Autodesk Fusion 360 part; units mm, degrees
(part 13 of 24)
  arc A3081 (7.8145, 16.0591) -> (7.8145, 16.3766) centre (7.8145, 16.2179) ccw
  arc A3082 (12.5666, 11.6245) -> (12.2491, 11.6245) centre (12.4078, 11.6245) ccw
  line L1039 (15.6337, 7.0391) -> (14.6591, 8.0137)
  line L1040 (12.4079, 11.6245) -> (12.259, 11.9839)
  arc A3083 (3.7529, 15.8555) -> (3.4354, 15.8555) centre (3.5941, 15.8555) ccw
  line L1041 (10.4521, 11.0249) -> (10.4521, 8.6955)
  arc A3084 (10.6108, 11.0249) -> (10.2934, 11.0249) centre (10.4521, 11.0249) ccw
  arc A3085 (10.4543, 8.2753) -> (10.7476, 8.3968) centre (10.601, 8.3361) ccw
  arc A3086 (72.6868, 22.0663) -> (72.6868, 22.3838) centre (72.6868, 22.2251) ccw
  arc A3087 (5.6955, 13.5954) -> (5.6955, 13.9129) centre (5.6955, 13.7542) ccw
  arc A3088 (14.3009, 32.0866) -> (14.3009, 32.404) centre (14.3009, 32.2453) ccw
  arc A3089 (56.8579, 22.3838) -> (56.8579, 22.0663) centre (56.8579, 22.2251) ccw
  arc A3090 (15.3797, 3.6512) -> (15.3797, 3.9687) centre (15.3797, 3.81) ccw
  arc A3091 (7.2149, 14.1034) -> (7.2149, 14.4208) centre (7.2149, 14.2621) ccw
  arc A3092 (14.5539, 2.2416) -> (14.5539, 2.5591) centre (14.5539, 2.4004) ccw
  arc A3093 (4.4645, 16.8846) -> (4.4645, 16.5671) centre (4.4645, 16.7259) ccw
  arc A3094 (15.7924, 7.0391) -> (15.4749, 7.0391) centre (15.6337, 7.0391) ccw
  arc A3095 (14.4417, 2.5126) -> (14.6662, 2.288) centre (14.554, 2.4003) ccw
  arc A3096 (13.8113, 3.81) -> (14.1288, 3.81) centre (13.9701, 3.81) ccw
  arc A3097 (13.8113, 2.4003) -> (14.1288, 2.4003) centre (13.9701, 2.4003) ccw
  line L1042 (13.6391, 32.2453) -> (14.3009, 32.2453)
  arc A3098 (6.2035, 16.3766) -> (6.2035, 16.0591) centre (6.2035, 16.2179) ccw
  line L1043 (3.5941, 14.6245) -> (4.4645, 13.7541)
  arc A3099 (12.1476, 5.6609) -> (12.465, 5.6609) centre (12.3063, 5.6609) ccw
  line L1044 (10.4521, 8.6955) -> (10.601, 8.3361)
  arc A3100 (44.8038, 14.6194) -> (44.5105, 14.7409) centre (44.6572, 14.6802) ccw
  arc A3101 (44.6251, 14.2194) -> (44.3076, 14.2194) centre (44.4664, 14.2194) ccw
  line L1045 (13.6893, 8.0137) -> (12.4079, 9.2951)
  line L1046 (12.5603, 3.2261) -> (13.3861, 2.4003)
  arc A3102 (12.2612, 11.5638) -> (12.5546, 11.6853) centre (12.4079, 11.6246) ccw
  line L1047 (13.0668, 4.9004) -> (12.5603, 4.3939)
  arc A3103 (45.5314, 15.077) -> (45.4099, 15.3704) centre (45.4706, 15.2237) ccw
  arc A3104 (3.4354, 14.6245) -> (3.7529, 14.6245) centre (3.5941, 14.6245) ccw
  line L1048 (44.4663, 13.7206) -> (44.6572, 13.2598)
  arc A3105 (13.6893, 8.1724) -> (13.6893, 7.8549) centre (13.6893, 8.0137) ccw
  arc A3106 (14.7714, 8.126) -> (14.5469, 7.9014) centre (14.6592, 8.0137) ccw
  arc A3107 (12.2491, 9.2951) -> (12.5666, 9.2951) centre (12.4078, 9.2951) ccw
  arc A3108 (6.2035, 14.4208) -> (6.2035, 14.1034) centre (6.2035, 14.2621) ccw
  line L1049 (3.5941, 15.8555) -> (3.5941, 14.6245)
  arc A3109 (8.1132, 15.9224) -> (8.2347, 16.2157) centre (8.1739, 16.0691) ccw
  arc A3110 (6.0912, 16.1056) -> (6.3157, 16.3302) centre (6.2035, 16.2179) ccw
  line L1050 (7.8145, 16.2179) -> (6.2035, 16.2179)
  arc A3111 (4.3523, 13.6418) -> (4.5768, 13.8664) centre (4.4646, 13.7541) ccw
  arc A3112 (12.5202, 9.4073) -> (12.2956, 9.1828) centre (12.4079, 9.2951) ccw
  arc A3113 (12.1468, 11.8717) -> (12.3713, 12.0962) centre (12.2591, 11.984) ccw
  arc A3114 (14.6591, 7.8549) -> (14.6591, 8.1724) centre (14.6591, 8.0137) ccw
  arc A3115 (7.8753, 16.3646) -> (7.7538, 16.0712) centre (7.8146, 16.2179) ccw
  arc A3116 (4.5768, 16.6136) -> (4.3523, 16.8382) centre (4.4645, 16.7259) ccw
  arc A3117 (10.3398, 10.9127) -> (10.5644, 11.1372) centre (10.4521, 11.025) ccw
  arc A3118 (5.6955, 16.5671) -> (5.6955, 16.8846) centre (5.6955, 16.7259) ccw
  line L1051 (14.6591, 8.0137) -> (13.6893, 8.0137)
  arc A3119 (5.5832, 13.8664) -> (5.8077, 13.6418) centre (5.6954, 13.7541) ccw
  arc A3120 (44.3076, 13.7206) -> (44.6251, 13.7206) centre (44.4664, 13.7206) ccw
  arc A3121 (44.3196, 14.2801) -> (44.613, 14.1586) centre (44.4663, 14.2193) ccw
  line L1052 (5.6955, 16.7259) -> (4.4645, 16.7259)
  arc A3122 (3.4818, 15.9677) -> (3.7064, 15.7432) centre (3.5941, 15.8554) ccw
  line L1053 (12.259, 11.9839) -> (11.9839, 12.259)
  arc A3123 (3.7064, 14.7368) -> (3.4818, 14.5123) centre (3.5941, 14.6246) ccw
  line L1054 (45.4706, 15.2237) -> (45.0098, 15.0328)
  arc A3124 (12.4057, 12.0447) -> (12.1124, 11.9232) centre (12.2591, 11.984) ccw
  arc A3125 (12.4016, 3.81) -> (12.719, 3.81) centre (12.5603, 3.81) ccw
  arc A3126 (14.1287, 3.81) -> (13.8112, 3.81) centre (13.97, 3.81) ccw
  line L1055 (12.5603, 3.81) -> (13.97, 3.81)
  line L1056 (5.6955, 13.7541) -> (6.2035, 14.2621)
  arc A3127 (5.8077, 16.8382) -> (5.5832, 16.6136) centre (5.6954, 16.7259) ccw
  line L1057 (12.3063, 5.6609) -> (13.0668, 4.9004)
  line L1058 (12.5603, 4.3939) -> (12.5603, 3.81)
  line L1059 (6.2035, 14.2621) -> (7.2149, 14.2621)
  line L1060 (8.1739, 16.069) -> (7.8145, 16.2179)
  arc A3128 (6.3157, 14.1498) -> (6.0912, 14.3744) centre (6.2035, 14.2621) ccw
  line L1061 (44.6572, 13.2598) -> (44.7421, 13.1749)
  line L1062 (10.601, 8.3361) -> (12.3063, 6.6307)
  arc A3129 (44.5105, 13.1991) -> (44.8038, 13.3206) centre (44.6572, 13.2599) ccw
  arc A3130 (10.2934, 8.6955) -> (10.6108, 8.6955) centre (10.4521, 8.6955) ccw
  line L1063 (11.9839, 12.259) -> (8.1739, 16.069)
  arc A3131 (12.4016, 3.2261) -> (12.719, 3.2261) centre (12.5603, 3.2261) ccw
  line L1064 (4.4645, 16.7259) -> (3.5941, 15.8555)
  arc A3132 (15.5214, 6.9269) -> (15.746, 7.1514) centre (15.6337, 7.0391) ccw
  arc A3133 (13.577, 7.9014) -> (13.8015, 8.1259) centre (13.6893, 8.0137) ccw
  arc A3134 (12.5603, 3.9688) -> (12.5603, 3.6513) centre (12.5603, 3.81) ccw
  arc A3135 (46.8149, 13.7206) -> (47.1324, 13.7206) centre (46.9737, 13.7206) ccw
  arc A3136 (12.194, 6.5185) -> (12.4186, 6.743) centre (12.3063, 6.6308) ccw
  arc A3137 (44.7694, 13.3721) -> (44.5449, 13.1476) centre (44.6571, 13.2599) ccw
  arc A3138 (12.465, 6.6307) -> (12.1476, 6.6307) centre (12.3063, 6.6307) ccw
  arc A3139 (44.6298, 13.0626) -> (44.8544, 13.2872) centre (44.7421, 13.1749) ccw
  line L1065 (44.7421, 13.1749) -> (44.7421, 7.8557)
  arc A3140 (44.8028, 7.709) -> (44.6814, 8.0024) centre (44.7421, 7.8557) ccw
  arc A3141 (44.9008, 13.1749) -> (44.5834, 13.1749) centre (44.7421, 13.1749) ccw
  arc A3142 (45.9694, 15.0649) -> (45.9694, 15.3824) centre (45.9694, 15.2236) ccw
  arc A3143 (13.2738, 2.288) -> (13.4983, 2.5126) centre (13.3861, 2.4003) ccw
  arc A3144 (40.0108, 7.9016) -> (40.1089, 7.5996) centre (40.0599, 7.7506) ccw
  arc A3145 (46.5424, 15.1451) -> (46.3179, 14.9206) centre (46.4301, 15.0329) ccw
  line L1066 (44.6572, 14.6802) -> (44.4663, 14.2194)
  arc A3146 (44.6593, 7.9932) -> (44.7808, 7.6999) centre (44.7201, 7.8466) ccw
  arc A3147 (43.5919, 8.262) -> (43.4704, 7.9686) centre (43.5312, 8.1153) ccw
  arc A3148 (44.1192, 7.6999) -> (44.2407, 7.9932) centre (44.1799, 7.8466) ccw
  arc A3149 (13.179, 4.7881) -> (12.9545, 5.0126) centre (13.0668, 4.9003) ccw
  arc A3150 (43.5311, 7.9565) -> (43.5311, 8.274) centre (43.5311, 8.1152) ccw
  arc A3151 (46.6706, 14.5679) -> (46.8951, 14.7924) centre (46.7829, 14.6801) ccw
  line L1067 (46.4302, 15.0328) -> (45.9694, 15.2237)
  arc A3152 (46.0301, 15.3704) -> (45.9086, 15.077) centre (45.9694, 15.2237) ccw
  line L1068 (45.9694, 15.2237) -> (45.4706, 15.2237)
  arc A3153 (46.9295, 14.7409) -> (46.6362, 14.6194) centre (46.7828, 14.6801) ccw
  arc A3154 (12.719, 4.3939) -> (12.4016, 4.3939) centre (12.5603, 4.3939) ccw
  line L1069 (12.5603, 3.81) -> (12.5603, 3.2261)
  arc A3155 (45.4706, 15.3824) -> (45.4706, 15.0649) centre (45.4706, 15.2236) ccw
  arc A3156 (47.1324, 14.2194) -> (46.8149, 14.2194) centre (46.9737, 14.2194) ccw
  arc A3157 (44.5834, 7.8557) -> (44.9008, 7.8557) centre (44.7421, 7.8557) ccw
  arc A3158 (12.6726, 3.3383) -> (12.448, 3.1138) centre (12.5603, 3.2261) ccw
  arc A3159 (13.97, 3.6513) -> (13.97, 3.9688) centre (13.97, 3.81) ccw
  line L1070 (46.9737, 14.2194) -> (46.7828, 14.6802)
  arc A3160 (46.3694, 14.8862) -> (46.4909, 15.1795) centre (46.4301, 15.0328) ccw
  arc A3161 (44.5449, 14.7924) -> (44.7694, 14.5679) centre (44.6571, 14.6802) ccw
  line L1071 (44.72, 7.8465) -> (44.45, 7.5765)
  line L1072 (44.7421, 7.8557) -> (44.72, 7.8465)
  line L1073 (44.4663, 14.2194) -> (44.4663, 13.7206)
  line L1074 (45.0098, 15.0328) -> (44.6572, 14.6802)
  line L1075 (39.6555, 7.5028) -> (39.4872, 7.3345)
  line L1076 (46.7828, 14.6802) -> (46.4302, 15.0328)
  arc A3162 (44.613, 13.7814) -> (44.3196, 13.6599) centre (44.4663, 13.7206) ccw
  arc A3163 (13.97, 3.6512) -> (13.97, 3.9687) centre (13.97, 3.81) ccw
  arc A3164 (12.4186, 5.7731) -> (12.194, 5.5486) centre (12.3063, 5.6609) ccw
  line L1077 (40.2861, 7.8241) -> (40.0599, 7.7506)
  line L1078 (46.9737, 13.7206) -> (46.9737, 14.2194)
  arc A3165 (41.6181, 7.5092) -> (41.8426, 7.2846) centre (41.7303, 7.3969) ccw
  arc A3166 (45.1221, 14.9206) -> (44.8976, 15.1451) centre (45.0099, 15.0328) ccw
  arc A3167 (39.375, 7.4468) -> (39.5995, 7.2223) centre (39.4873, 7.3346) ccw
  arc A3168 (12.719, 3.81) -> (12.4016, 3.81) centre (12.5603, 3.81) ccw
  arc A3169 (13.8112, 3.81) -> (14.1287, 3.81) centre (13.97, 3.81) ccw
  arc A3170 (40.9691, 7.6673) -> (41.0187, 7.9809) centre (40.9939, 7.8241) ccw
  line L1079 (43.5311, 8.1153) -> (42.8289, 8.1153)
  arc A3171 (42.8896, 7.9686) -> (42.7681, 8.262) centre (42.8289, 8.1153) ccw
  line L1080 (13.97, 3.81) -> (12.5603, 3.81)
  arc A3172 (44.9491, 15.1795) -> (45.0706, 14.8862) centre (45.0099, 15.0328) ccw
  arc A3173 (42.2923, 7.7343) -> (42.0678, 7.9588) centre (42.18, 7.8466) ccw
  arc A3174 (12.9545, 4.7881) -> (13.179, 5.0126) centre (13.0668, 4.9003) ccw
  arc A3175 (40.64, 8.02) -> (40.64, 7.7025) centre (40.64, 7.8613) ccw
  line L1081 (41.2201, 7.7506) -> (40.9939, 7.8241)
  arc A3176 (12.448, 4.5062) -> (12.6726, 4.2817) centre (12.5603, 4.394) ccw
  line L1082 (40.9939, 7.8241) -> (40.7589, 7.8613)
  arc A3177 (46.827, 14.1586) -> (47.1204, 14.2801) centre (46.9737, 14.2194) ccw
  arc A3178 (41.7368, 7.615) -> (41.5123, 7.3905) centre (41.6246, 7.5027) ccw
  arc A3179 (12.5603, 3.9687) -> (12.5603, 3.6512) centre (12.5603, 3.81) ccw
  arc A3180 (39.7677, 7.3905) -> (39.5432, 7.615) centre (39.6555, 7.5028) ccw
  line L1083 (42.8289, 8.1153) -> (42.18, 7.8465)
  arc A3181 (40.7987, 7.8613) -> (40.4812, 7.8613) centre (40.6399, 7.8613) ccw
  arc A3182 (41.5312, 7.3743) -> (41.7179, 7.6312) centre (41.6246, 7.5027) ccw
  arc A3183 (41.36, 7.5011) -> (41.5042, 7.784) centre (41.4321, 7.6425) ccw
  arc A3184 (40.7988, 7.8613) -> (40.4813, 7.8613) centre (40.6401, 7.8613) ccw
  arc A3185 (40.64, 6.1913) -> (40.64, 6.5088) centre (40.64, 6.3501) ccw
  arc A3186 (39.2416, 7.2665) -> (39.4984, 7.0799) centre (39.37, 7.1732) ccw
  arc A3187 (34.6723, 7.7343) -> (34.4478, 7.9588) centre (34.5601, 7.8466) ccw
  arc A3188 (41.043, 7.9751) -> (40.9448, 7.6731) centre (40.9939, 7.8241) ccw
  arc A3189 (38.2438, 8.0181) -> (38.1941, 7.7045) centre (38.2189, 7.8613) ccw
  arc A3190 (41.2922, 7.892) -> (41.1481, 7.6091) centre (41.2202, 7.7506) ccw
  arc A3191 (35.2696, 7.9686) -> (35.1481, 8.262) centre (35.2088, 8.1153) ccw
  line L1084 (40.0599, 7.7506) -> (39.8479, 7.6426)
  arc A3192 (42.8289, 8.274) -> (42.8289, 7.9565) centre (42.8289, 8.1152) ccw
  line L1085 (35.9111, 8.1153) -> (35.2089, 8.1153)
  arc A3193 (38.1, 7.7025) -> (38.1, 8.02) centre (38.1, 7.8613) ccw
  arc A3194 (38.9912, 7.3743) -> (39.1779, 7.6312) centre (39.0846, 7.5028) ccw
  line L1086 (37.7461, 7.8241) -> (37.5199, 7.7506)
  arc A3195 (40.5211, 8.02) -> (40.5211, 7.7025) centre (40.5211, 7.8613) ccw
  arc A3196 (37.2358, 7.784) -> (37.38, 7.5011) centre (37.3079, 7.6425) ccw
  line L1087 (41.7304, 7.3969) -> (41.6245, 7.5028)
  arc A3197 (38.2189, 7.7025) -> (38.2189, 8.02) centre (38.2189, 7.8613) ccw
  line L1088 (37.1155, 7.5028) -> (37.0096, 7.3969)
  arc A3198 (41.6181, 7.2846) -> (41.8426, 7.5092) centre (41.7304, 7.3969) ccw
  line L1089 (39.37, 7.1732) -> (39.2528, 7.3345)
  arc A3199 (38.1, 8.02) -> (38.1, 7.7025) centre (38.1, 7.8613) ccw
  arc A3200 (35.2089, 8.274) -> (35.2089, 7.9565) centre (35.2089, 8.1152) ccw
  line L1090 (39.4872, 7.3345) -> (39.37, 7.1732)
  arc A3201 (37.0221, 7.6312) -> (37.2088, 7.3743) centre (37.1155, 7.5028) ccw
  line L1091 (40.64, 7.8613) -> (40.64, 6.35)
  arc A3202 (38.6311, 7.5996) -> (38.7292, 7.9016) centre (38.6802, 7.7506) ccw
  arc A3203 (40.7838, 8.0181) -> (40.7341, 7.7045) centre (40.7589, 7.8613) ccw
  arc A3204 (36.8973, 7.2846) -> (37.1219, 7.5092) centre (37.0096, 7.3969) ccw
  line L1092 (44.45, 7.5765) -> (44.18, 7.8465)
  line L1093 (39.8479, 7.6426) -> (39.6555, 7.5028)
  arc A3205 (40.1319, 7.6091) -> (39.9878, 7.892) centre (40.0599, 7.7506) ccw
  arc A3206 (40.64, 7.7025) -> (40.64, 8.02) centre (40.64, 7.8613) ccw
  arc A3207 (39.6157, 7.2412) -> (39.3588, 7.4279) centre (39.4873, 7.3346) ccw
  arc A3208 (40.7589, 7.7025) -> (40.7589, 8.02) centre (40.7589, 7.8613) ccw
  line L1094 (40.64, 7.8613) -> (40.5211, 7.8613)
  line L1095 (41.4321, 7.6426) -> (41.2201, 7.7506)
  arc A3209 (39.9412, 7.5141) -> (39.7546, 7.771) centre (39.8479, 7.6425) ccw
  arc A3210 (40.4813, 6.35) -> (40.7988, 6.35) centre (40.6401, 6.35) ccw
  arc A3211 (44.3377, 7.4643) -> (44.5623, 7.6888) centre (44.45, 7.5766) ccw
  line L1096 (41.6245, 7.5028) -> (41.4321, 7.6426)
  arc A3212 (44.3377, 7.6888) -> (44.5623, 7.4643) centre (44.45, 7.5766) ccw
  arc A3213 (40.64, 6.5088) -> (40.64, 6.1913) centre (40.64, 6.3501) ccw
  line L1097 (40.7589, 7.8613) -> (40.64, 7.8613)
  line L1098 (37.9811, 7.8613) -> (37.7461, 7.8241)
  line L1099 (40.5211, 7.8613) -> (40.2861, 7.8241)
  arc A3214 (44.8323, 7.7343) -> (44.6078, 7.9588) centre (44.72, 7.8466) ccw
  arc A3215 (41.5254, 7.771) -> (41.3388, 7.5141) centre (41.4321, 7.6426) ccw
  line L1100 (38.1, 6.35) -> (38.1, 7.8613)
  line L1101 (40.64, 6.35) -> (40.64, 7.8613)
  arc A3216 (40.3352, 7.6731) -> (40.237, 7.9751) centre (40.2861, 7.8241) ccw
  arc A3217 (42.1193, 7.9932) -> (42.2408, 7.6999) centre (42.18, 7.8465) ccw
  arc A3218 (41.1711, 7.5996) -> (41.2692, 7.9016) centre (41.2202, 7.7506) ccw
  line L1102 (44.18, 7.8465) -> (43.5311, 8.1153)
  arc A3219 (40.5459, 7.7045) -> (40.4962, 8.0181) centre (40.5211, 7.8613) ccw
  arc A3220 (44.2922, 7.9588) -> (44.0677, 7.7343) centre (44.18, 7.8465) ccw
  arc A3221 (39.7758, 7.784) -> (39.92, 7.5011) centre (39.8479, 7.6426) ccw
  arc A3222 (34.1777, 7.6888) -> (34.4023, 7.4643) centre (34.29, 7.5765) ccw
  arc A3223 (40.2613, 7.9809) -> (40.3109, 7.6673) centre (40.2861, 7.8241) ccw
  line L1103 (37.5199, 7.7506) -> (37.3079, 7.6426)
  arc A3224 (39.5621, 7.6312) -> (39.7488, 7.3743) centre (39.6555, 7.5028) ccw
  line L1104 (34.56, 7.8465) -> (34.29, 7.5765)
  arc A3225 (40.4812, 6.35) -> (40.7987, 6.35) centre (40.6399, 6.35) ccw
  line L1105 (42.18, 7.8465) -> (41.7304, 7.3969)
  arc A3226 (38.9854, 7.771) -> (38.7988, 7.5141) centre (38.8921, 7.6425) ccw
  arc A3227 (34.4993, 7.9932) -> (34.6208, 7.6999) centre (34.5601, 7.8466) ccw
  arc A3228 (37.4708, 7.9016) -> (37.5689, 7.5996) centre (37.5199, 7.7506) ccw
  arc A3229 (36.4992, 7.6999) -> (36.6207, 7.9932) centre (36.5599, 7.8466) ccw
  arc A3230 (38.7522, 7.892) -> (38.6081, 7.6091) centre (38.6802, 7.7505) ccw
  arc A3231 (38.4291, 7.6673) -> (38.4787, 7.9809) centre (38.4539, 7.8241) ccw
  arc A3232 (36.8973, 7.5092) -> (37.1219, 7.2846) centre (37.0096, 7.3969) ccw
  arc A3233 (37.5919, 7.6091) -> (37.4478, 7.892) centre (37.5199, 7.7506) ccw
  arc A3234 (39.1968, 7.615) -> (38.9723, 7.3905) centre (39.0846, 7.5028) ccw
  line L1106 (38.2189, 7.8613) -> (38.1, 7.8613)
  line L1107 (29.21, 15.2835) -> (29.48, 15.0135)
  arc A3235 (37.7213, 7.9809) -> (37.7709, 7.6673) centre (37.7461, 7.8241) ccw
  arc A3236 (29.3678, 14.9012) -> (29.5923, 15.1257) centre (29.4801, 15.0135) ccw
  line L1108 (31.6665, 7.493) -> (30.9534, 7.493)
  line L1109 (38.1, 7.8613) -> (38.1, 6.35)
  arc A3237 (38.503, 7.9751) -> (38.4048, 7.6731) centre (38.4539, 7.8241) ccw
  arc A3238 (35.9719, 8.262) -> (35.8504, 7.9686) centre (35.9112, 8.1153) ccw
  arc A3239 (37.9811, 8.02) -> (37.9811, 7.7025) centre (37.9811, 7.8613) ccw
  line L1110 (26.4, 15.0135) -> (26.67, 15.2835)
  arc A3240 (25.6904, 14.8914) -> (25.8119, 14.598) centre (25.7512, 14.7447) ccw
  arc A3241 (30.0681, 14.598) -> (30.1896, 14.8914) centre (30.1288, 14.7447) ccw
  arc A3242 (37.9413, 6.35) -> (38.2588, 6.35) centre (38.1, 6.35) ccw
  arc A3243 (39.3812, 7.4279) -> (39.1243, 7.2412) centre (39.2527, 7.3346) ccw
  arc A3244 (37.4012, 7.5141) -> (37.2146, 7.771) centre (37.3079, 7.6425) ccw
  line L1111 (30.1289, 14.7447) -> (30.8311, 14.7447)
  arc A3245 (38.1, 6.5088) -> (38.1, 6.1913) centre (38.1, 6.3501) ccw
  arc A3246 (23.8907, 15.2687) -> (24.1153, 15.0442) centre (24.003, 15.1565) ccw
  arc A3247 (24.2423, 15.3957) -> (24.0177, 15.1712) centre (24.13, 15.2835) ccw
  arc A3248 (34.1777, 7.4643) -> (34.4023, 7.6888) centre (34.29, 7.5765) ccw
  line L1112 (38.4539, 7.8241) -> (38.2189, 7.8613)
  arc A3249 (39.1405, 7.2223) -> (39.365, 7.4468) centre (39.2528, 7.3346) ccw
  arc A3250 (26.7823, 15.1712) -> (26.5577, 15.3957) centre (26.67, 15.2835) ccw
  line L1113 (24.13, 15.2835) -> (24.4, 15.0135)
  line L1114 (25.0489, 14.7447) -> (25.7511, 14.7447)
  line L1115 (39.2528, 7.3345) -> (39.0845, 7.5028)
  arc A3251 (38.2588, 7.8613) -> (37.9413, 7.8613) centre (38.1, 7.8613) ccw
  arc A3252 (25.0489, 14.9034) -> (25.0489, 14.586) centre (25.0489, 14.7447) ccw
  arc A3253 (29.3223, 15.1712) -> (29.0977, 15.3957) centre (29.21, 15.2835) ccw
  arc A3254 (26.2877, 15.1257) -> (26.5122, 14.9012) centre (26.4, 15.0135) ccw
  line L1116 (39.0845, 7.5028) -> (38.8921, 7.6426)
  arc A3255 (29.3223, 15.3957) -> (29.0977, 15.1712) centre (29.21, 15.2834) ccw
  arc A3256 (38.2587, 7.8613) -> (37.9412, 7.8613) centre (38.0999, 7.8613) ccw
  line L1117 (25.7511, 14.7447) -> (26.4, 15.0135)
  line L1118 (37.0096, 7.3969) -> (36.56, 7.8465)
  arc A3257 (29.5408, 15.1601) -> (29.4193, 14.8668) centre (29.4801, 15.0135) ccw
  arc A3258 (31.6665, 7.3342) -> (31.6665, 7.6517) centre (31.6665, 7.493) ccw
  arc A3259 (34.1322, 7.9588) -> (33.9077, 7.7343) centre (34.02, 7.8466) ccw
  line L1119 (36.56, 7.8465) -> (35.9111, 8.1153)
  line L1120 (34.29, 7.5765) -> (34.02, 7.8465)
  arc A3260 (38.1, 6.1913) -> (38.1, 6.5088) centre (38.1, 6.3501) ccw
  line L1121 (28.94, 15.0135) -> (29.21, 15.2835)
  arc A3261 (37.7952, 7.6731) -> (37.697, 7.9751) centre (37.7461, 7.8241) ccw
  arc A3262 (37.9412, 6.35) -> (38.2587, 6.35) centre (38.0999, 6.35) ccw
  arc A3263 (35.9111, 7.9565) -> (35.9111, 8.274) centre (35.9111, 8.1152) ccw
  line L1122 (38.1, 7.8613) -> (37.9811, 7.8613)
  arc A3264 (37.2277, 7.3905) -> (37.0032, 7.615) centre (37.1155, 7.5028) ccw
  line L1123 (35.2089, 8.1153) -> (34.56, 7.8465)
  arc A3265 (38.0059, 7.7045) -> (37.9562, 8.0181) centre (37.9811, 7.8613) ccw
  line L1124 (38.6801, 7.7506) -> (38.4539, 7.8241)
  arc A3266 (36.6722, 7.9588) -> (36.4477, 7.7343) centre (36.56, 7.8466) ccw
  line L1125 (38.8921, 7.6426) -> (38.6801, 7.7506)
  line L1126 (37.3079, 7.6426) -> (37.1155, 7.5028)
  arc A3267 (38.82, 7.5011) -> (38.9642, 7.784) centre (38.8921, 7.6425) ccw
  arc A3268 (39.2416, 7.0799) -> (39.4984, 7.2665) centre (39.37, 7.1732) ccw
  line L1127 (29.48, 15.0135) -> (30.1289, 14.7447)
  arc A3269 (24.2423, 15.1712) -> (24.0177, 15.3957) centre (24.13, 15.2835) ccw
  arc A3270 (31.5542, 7.6052) -> (31.7787, 7.3807) centre (31.6665, 7.493) ccw
  line L1128 (40.0599, 15.1094) -> (40.2861, 15.0359)
  arc A3271 (29.0007, 14.8668) -> (28.8792, 15.1601) centre (28.94, 15.0135) ccw
  line L1129 (39.8479, 15.2174) -> (40.0599, 15.1094)
  line L1130 (37.7489, 14.7447) -> (38.4511, 14.7447)
  arc A3272 (32.7296, 7.9686) -> (32.6081, 8.262) centre (32.6689, 8.1153) ccw
  arc A3273 (27.5889, 14.9034) -> (27.5889, 14.586) centre (27.5889, 14.7447) ccw
  line L1131 (24.003, 15.1565) -> (24.13, 15.2835)
  line L1132 (32.02, 7.8465) -> (31.6665, 7.493)
  arc A3274 (24.1153, 14.5557) -> (23.8907, 14.3312) centre (24.003, 14.4435) ccw
  line L1133 (30.9534, 7.493) -> (24.003, 14.4434)
  arc A3275 (25.7511, 14.586) -> (25.7511, 14.9034) centre (25.7511, 14.7447) ccw
  arc A3276 (33.4319, 8.262) -> (33.3104, 7.9686) centre (33.3712, 8.1153) ccw
  line L1134 (27.5889, 14.7447) -> (28.2911, 14.7447)
  arc A3277 (23.8442, 14.4434) -> (24.1617, 14.4434) centre (24.003, 14.4434) ccw
  arc A3278 (40.237, 14.8849) -> (40.3352, 15.1869) centre (40.2861, 15.0359) ccw
  arc A3279 (33.3711, 7.9565) -> (33.3711, 8.274) centre (33.3711, 8.1152) ccw
  arc A3280 (34.0807, 14.8668) -> (33.9592, 15.1601) centre (34.02, 15.0135) ccw
  arc A3281 (33.9077, 15.1257) -> (34.1322, 14.9012) centre (34.02, 15.0135) ccw
  arc A3282 (32.1323, 7.7343) -> (31.9078, 7.9588) centre (32.0201, 7.8466) ccw
  arc A3283 (34.6208, 15.1601) -> (34.4993, 14.8668) centre (34.5601, 15.0135) ccw
  line L1135 (34.02, 7.8465) -> (33.3711, 8.1153)
  line L1136 (34.02, 15.0135) -> (34.29, 15.2835)
  line L1137 (24.4, 15.0135) -> (25.0489, 14.7447)
  arc A3284 (26.8278, 14.9012) -> (27.0523, 15.1257) centre (26.9401, 15.0135) ccw
  arc A3285 (30.1289, 14.9034) -> (30.1289, 14.586) centre (30.1289, 14.7447) ccw
  arc A3286 (28.2911, 14.586) -> (28.2911, 14.9034) centre (28.2911, 14.7447) ccw
  arc A3287 (28.2304, 14.8914) -> (28.3519, 14.598) centre (28.2911, 14.7447) ccw
  arc A3288 (39.6619, 15.5753) -> (39.4373, 15.3508) centre (39.5496, 15.4631) ccw
  arc A3289 (34.4023, 15.3957) -> (34.1777, 15.1712) centre (34.29, 15.2834) ccw
  arc A3290 (26.4607, 14.8668) -> (26.3392, 15.1601) centre (26.4, 15.0134) ccw
  arc A3291 (26.7823, 15.3957) -> (26.5577, 15.1712) centre (26.67, 15.2835) ccw
  line L1138 (36.83, 15.2835) -> (37.1, 15.0135)
  arc A3292 (33.3104, 14.8914) -> (33.4319, 14.598) centre (33.3712, 14.7447) ccw
  line L1139 (36.56, 15.0135) -> (36.83, 15.2835)
  arc A3293 (31.3677, 15.1257) -> (31.5922, 14.9012) centre (31.4799, 15.0135) ccw
  arc A3294 (32.6689, 8.274) -> (32.6689, 7.9565) centre (32.6689, 8.1152) ccw
  arc A3295 (39.1607, 14.8668) -> (39.0392, 15.1601) centre (39.1, 15.0135) ccw
  arc A3296 (35.2089, 14.9034) -> (35.2089, 14.586) centre (35.2089, 14.7447) ccw
  arc A3297 (24.4608, 15.1601) -> (24.3393, 14.8668) centre (24.4001, 15.0135) ccw
  arc A3298 (27.0008, 15.1601) -> (26.8793, 14.8668) centre (26.9401, 15.0135) ccw
  arc A3299 (31.9593, 7.9932) -> (32.0808, 7.6999) centre (32.0201, 7.8466) ccw
  arc A3300 (27.5281, 14.598) -> (27.6496, 14.8914) centre (27.5889, 14.7447) ccw
  arc A3301 (30.8311, 14.586) -> (30.8311, 14.9034) centre (30.8311, 14.7447) ccw
  line L1140 (39.6555, 15.3572) -> (39.8479, 15.2174)
  arc A3302 (30.9534, 7.6517) -> (30.9534, 7.3342) centre (30.9534, 7.493) ccw
  line L1141 (24.003, 14.4434) -> (24.003, 15.1565)
  arc A3303 (39.9878, 14.968) -> (40.1319, 15.2509) centre (40.0599, 15.1094) ccw
  line L1142 (26.94, 15.0135) -> (27.5889, 14.7447)
  arc A3304 (36.9423, 15.1712) -> (36.7177, 15.3957) centre (36.83, 15.2835) ccw
  arc A3305 (37.7489, 14.9034) -> (37.7489, 14.586) centre (37.7489, 14.7447) ccw
  arc A3306 (39.92, 15.3589) -> (39.7758, 15.076) centre (39.8479, 15.2175) ccw
  arc A3307 (28.8277, 15.1257) -> (29.0522, 14.9012) centre (28.94, 15.0135) ccw
  arc A3308 (33.9592, 7.6999) -> (34.0807, 7.9932) centre (34.02, 7.8466) ccw
  arc A3309 (24.1617, 15.1565) -> (23.8442, 15.1565) centre (24.003, 15.1565) ccw
  line L1143 (26.67, 15.2835) -> (26.94, 15.0135)
  arc A3310 (30.8412, 7.3807) -> (31.0657, 7.6053) centre (30.9534, 7.493) ccw
  line L1144 (28.2911, 14.7447) -> (28.94, 15.0135)
  line L1145 (32.6689, 8.1153) -> (32.02, 7.8465)
  arc A3311 (39.7488, 15.4857) -> (39.5621, 15.2288) centre (39.6555, 15.3573) ccw
  line L1146 (33.3711, 8.1153) -> (32.6689, 8.1153)
  arc A3312 (24.2878, 14.9012) -> (24.5123, 15.1257) centre (24.4001, 15.0135) ccw
  arc A3313 (24.9881, 14.598) -> (25.1096, 14.8914) centre (25.0489, 14.7447) ccw
  line L1147 (31.75, 15.2835) -> (32.02, 15.0135)
  line L1148 (35.9111, 14.7447) -> (36.56, 15.0135)
  arc A3314 (30.7704, 14.8914) -> (30.8919, 14.598) centre (30.8312, 14.7447) ccw
  line L1149 (32.02, 15.0135) -> (32.6689, 14.7447)
  arc A3315 (36.9878, 14.9012) -> (37.2123, 15.1257) centre (37.1001, 15.0135) ccw
  arc A3316 (32.6689, 14.9034) -> (32.6689, 14.586) centre (32.6689, 14.7447) ccw
  arc A3317 (31.5407, 14.8668) -> (31.4192, 15.1601) centre (31.4799, 15.0135) ccw
  line L1150 (39.5496, 15.4631) -> (39.6555, 15.3572)
  line L1151 (34.56, 15.0135) -> (35.2089, 14.7447)
  arc A3318 (36.4477, 15.1257) -> (36.6722, 14.9012) centre (36.56, 15.0135) ccw
  line L1152 (33.3711, 14.7447) -> (34.02, 15.0135)
  arc A3319 (31.8623, 15.3957) -> (31.6377, 15.1712) centre (31.75, 15.2835) ccw
  line L1153 (40.2861, 15.0359) -> (40.5211, 14.9987)
  arc A3320 (36.9423, 15.3957) -> (36.7177, 15.1712) centre (36.83, 15.2834) ccw
  arc A3321 (35.9111, 14.586) -> (35.9111, 14.9034) centre (35.9111, 14.7447) ccw
  arc A3322 (32.6081, 14.598) -> (32.7296, 14.8914) centre (32.6689, 14.7447) ccw
  line L1154 (35.2089, 14.7447) -> (35.9111, 14.7447)
  line L1155 (31.48, 15.0135) -> (31.75, 15.2835)
  arc A3323 (32.0808, 15.1601) -> (31.9593, 14.8668) centre (32.0201, 15.0134) ccw
  line L1156 (39.1, 15.0135) -> (39.5496, 15.4631)
  arc A3324 (38.9877, 15.1257) -> (39.2122, 14.9012) centre (39.1, 15.0135) ccw
  arc A3325 (39.5432, 15.245) -> (39.7677, 15.4695) centre (39.6555, 15.3573) ccw
  arc A3326 (37.6881, 14.598) -> (37.8096, 14.8914) centre (37.7489, 14.7447) ccw
  arc A3327 (31.8623, 15.1712) -> (31.6377, 15.3957) centre (31.75, 15.2835) ccw
  arc A3328 (31.9078, 14.9012) -> (32.1323, 15.1257) centre (32.0201, 15.0135) ccw
  line L1157 (40.64, 14.9987) -> (40.64, 16.51)
  arc A3329 (41.8896, 15.9789) -> (42.1916, 15.8808) centre (42.0406, 15.9299) ccw
  arc A3330 (38.3904, 14.8914) -> (38.5119, 14.598) centre (38.4511, 14.7447) ccw
  arc A3331 (41.5123, 15.4695) -> (41.7368, 15.245) centre (41.6246, 15.3573) ccw
  arc A3332 (39.7546, 15.089) -> (39.9412, 15.3458) centre (39.8479, 15.2174) ccw
  arc A3333 (38.4511, 14.586) -> (38.4511, 14.9034) centre (38.4511, 14.7447) ccw
  arc A3334 (42.1513, 16.3513) -> (42.1513, 16.6688) centre (42.1513, 16.51) ccw
  line L1158 (30.8311, 14.7447) -> (31.48, 15.0135)
  arc A3335 (40.4962, 14.8419) -> (40.5459, 15.1555) centre (40.5211, 14.9987) ccw
  arc A3336 (40.5211, 15.1574) -> (40.5211, 14.84) centre (40.5211, 14.9987) ccw
  line L1159 (41.7928, 15.5255) -> (41.9326, 15.7179)
  arc A3337 (35.8504, 14.8914) -> (35.9719, 14.598) centre (35.9112, 14.7447) ccw
  line L1160 (42.1141, 16.1561) -> (42.1513, 16.3911)
  arc A3338 (42.31, 16.6289) -> (41.9925, 16.6289) centre (42.1513, 16.6289) ccw
  line L1161 (40.64, 16.51) -> (40.64, 14.9987)
  arc A3339 (39.6619, 15.3508) -> (39.4373, 15.5753) centre (39.5496, 15.4631) ccw
  line L1162 (42.1513, 16.51) -> (42.1513, 16.6289)
  line L1163 (34.29, 15.2835) -> (34.56, 15.0135)
  arc A3340 (33.3711, 14.586) -> (33.3711, 14.9034) centre (33.3711, 14.7447) ccw
  arc A3341 (36.6207, 14.8668) -> (36.4992, 15.1601) centre (36.56, 15.0134) ccw
  line L1164 (37.1, 15.0135) -> (37.7489, 14.7447)
  line L1165 (32.6689, 14.7447) -> (33.3711, 14.7447)
  arc A3342 (37.1608, 15.1601) -> (37.0393, 14.8668) centre (37.1, 15.0134) ccw
  arc A3343 (35.1481, 14.598) -> (35.2696, 14.8914) centre (35.2088, 14.7447) ccw
  arc A3344 (40.1089, 15.2604) -> (40.0108, 14.9584) centre (40.0599, 15.1094) ccw
  line L1166 (38.4511, 14.7447) -> (39.1, 15.0135)
  arc A3345 (34.4478, 14.9012) -> (34.6723, 15.1257) centre (34.5601, 15.0135) ccw
  arc A3346 (40.64, 16.6688) -> (40.64, 16.3513) centre (40.64, 16.51) ccw
  line L1167 (41.2201, 15.1094) -> (41.4321, 15.2174)
  arc A3347 (34.4023, 15.1712) -> (34.1777, 15.3957) centre (34.29, 15.2835) ccw
  arc A3348 (41.9925, 16.51) -> (42.31, 16.51) centre (42.1513, 16.51) ccw
  arc A3349 (40.7987, 16.51) -> (40.4812, 16.51) centre (40.6399, 16.51) ccw
  arc A3350 (41.2692, 14.9584) -> (41.1711, 15.2604) centre (41.2202, 15.1094) ccw
  arc A3351 (40.4813, 16.51) -> (40.7988, 16.51) centre (40.6401, 16.51) ccw
  line L1168 (41.4321, 15.2174) -> (41.6245, 15.3572)
  arc A3352 (40.64, 16.6688) -> (40.64, 16.3513) centre (40.64, 16.51) ccw
  arc A3353 (40.4812, 16.51) -> (40.7987, 16.51) centre (40.6399, 16.51) ccw
  arc A3354 (40.64, 17.8625) -> (40.64, 18.18) centre (40.64, 18.0212) ccw
  arc A3355 (41.9925, 16.3911) -> (42.31, 16.3911) centre (42.1513, 16.3911) ccw
  arc A3356 (40.4812, 14.9987) -> (40.7987, 14.9987) centre (40.6399, 14.9987) ccw
  line L1169 (41.6245, 15.3572) -> (41.7928, 15.5255)
  arc A3357 (41.3388, 15.3458) -> (41.5254, 15.089) centre (41.4321, 15.2174) ccw
  arc A3358 (41.6643, 15.6188) -> (41.9212, 15.4321) centre (41.7927, 15.5255) ccw
  line L1170 (42.0406, 15.9299) -> (42.1141, 16.1561)
  line L1171 (40.9939, 15.0359) -> (41.2201, 15.1094)
  line L1172 (42.0406, 17.0901) -> (41.9326, 17.3021)
  arc A3359 (40.64, 16.6687) -> (40.64, 16.3512) centre (40.64, 16.5099) ccw
  line L1173 (40.2861, 17.9841) -> (40.0599, 17.9106)
  arc A3360 (40.3352, 17.8331) -> (40.237, 18.1351) centre (40.2861, 17.9841) ccw
  arc A3361 (39.7758, 17.944) -> (39.92, 17.6611) centre (39.8479, 17.8026) ccw
  line L1174 (42.1513, 16.51) -> (40.64, 16.51)
  arc A3362 (40.64, 15.1575) -> (40.64, 14.84) centre (40.64, 14.9988) ccw
  arc A3363 (41.9631, 16.8148) -> (42.2651, 16.913) centre (42.1141, 16.8639) ccw
  arc A3364 (39.9412, 17.6741) -> (39.7546, 17.931) centre (39.8479, 17.8025) ccw
  arc A3365 (39.4373, 17.6692) -> (39.6619, 17.4446) centre (39.5496, 17.5569) ccw
  arc A3366 (42.3081, 16.3662) -> (41.9945, 16.4159) centre (42.1513, 16.3911) ccw
  arc A3367 (42.1916, 17.1392) -> (41.8896, 17.0411) centre (42.0406, 17.0902) ccw
  arc A3368 (41.0187, 14.8791) -> (40.9691, 15.1927) centre (40.9939, 15.0359) ccw
  line L1175 (39.1, 18.0065) -> (38.4511, 18.2753)
  line L1176 (41.9326, 15.7179) -> (42.0406, 15.9299)
  arc A3369 (40.1319, 17.7691) -> (39.9878, 18.052) centre (40.0599, 17.9106) ccw
  arc A3370 (41.8041, 17.2088) -> (42.061, 17.3954) centre (41.9326, 17.3021) ccw
  arc A3371 (40.9448, 15.1869) -> (41.043, 14.8849) centre (40.9939, 15.0359) ccw
  line L1177 (40.5211, 18.0213) -> (40.2861, 17.9841)
  arc A3372 (40.7341, 15.1555) -> (40.7838, 14.8419) centre (40.7589, 14.9987) ccw
  arc A3373 (41.905, 15.4132) -> (41.6805, 15.6377) centre (41.7928, 15.5254) ccw
  arc A3374 (40.7988, 16.51) -> (40.4813, 16.51) centre (40.6401, 16.51) ccw
  line L1178 (40.64, 14.9987) -> (40.7589, 14.9987)
  arc A3375 (41.5042, 15.076) -> (41.36, 15.3589) centre (41.4321, 15.2175) ccw
  arc A3376 (42.1513, 16.3512) -> (42.1513, 16.6687) centre (42.1513, 16.5099) ccw
  line L1179 (42.1141, 16.8639) -> (42.0406, 17.0901)
  arc A3377 (42.061, 15.6246) -> (41.8041, 15.8112) centre (41.9326, 15.7179) ccw
  line L1180 (40.64, 16.51) -> (42.1513, 16.51)
  arc A3378 (41.9573, 16.1809) -> (42.2709, 16.1313) centre (42.1141, 16.1561) ccw
  line L1181 (40.5211, 14.9987) -> (40.64, 14.9987)
  arc A3379 (42.2709, 16.8887) -> (41.9573, 16.8391) centre (42.1141, 16.8639) ccw
  arc A3380 (42.2651, 16.107) -> (41.9631, 16.2052) centre (42.1141, 16.1561) ccw
  arc A3381 (41.9945, 16.6041) -> (42.3081, 16.6538) centre (42.1513, 16.629) ccw
  arc A3382 (40.7589, 14.84) -> (40.7589, 15.1575) centre (40.7589, 14.9988) ccw
  arc A3383 (40.64, 16.3512) -> (40.64, 16.6687) centre (40.64, 16.5099) ccw
  arc A3384 (40.4813, 14.9987) -> (40.7988, 14.9987) centre (40.6401, 14.9987) ccw
  line L1182 (42.1513, 16.6289) -> (42.1141, 16.8639)
  line L1183 (40.7589, 14.9987) -> (40.9939, 15.0359)
  arc A3385 (41.7179, 15.2288) -> (41.5312, 15.4857) centre (41.6246, 15.3573) ccw
  arc A3386 (40.64, 16.6687) -> (40.64, 16.3512) centre (40.64, 16.5099) ccw
  arc A3387 (40.3109, 15.1927) -> (40.2613, 14.8791) centre (40.2861, 15.0359) ccw
  arc A3388 (42.182, 15.8578) -> (41.8991, 16.0019) centre (42.0406, 15.9299) ccw
  arc A3389 (42.31, 16.51) -> (41.9925, 16.51) centre (42.1513, 16.51) ccw
  arc A3390 (40.7988, 16.51) -> (40.4813, 16.51) centre (40.6401, 16.51) ccw
  arc A3391 (40.64, 14.8399) -> (40.64, 15.1574) centre (40.64, 14.9986) ccw
  line L1184 (42.1513, 16.3911) -> (42.1513, 16.51)
  arc A3392 (41.1481, 15.2509) -> (41.2922, 14.968) centre (41.2202, 15.1094) ccw
  arc A3393 (41.7911, 15.79) -> (42.074, 15.6458) centre (41.9325, 15.7179) ccw
  arc A3394 (38.4511, 18.1165) -> (38.4511, 18.434) centre (38.4511, 18.2752) ccw
  arc A3395 (40.7838, 18.1781) -> (40.7341, 17.8645) centre (40.7589, 18.0213) ccw
  arc A3396 (37.2123, 17.8943) -> (36.9878, 18.1188) centre (37.1001, 18.0066) ccw
  line L1185 (39.6555, 17.6628) -> (39.5496, 17.5569)
  line L1186 (40.7589, 18.0213) -> (40.64, 18.0213)
  arc A3397 (37.7489, 18.434) -> (37.7489, 18.1165) centre (37.7489, 18.2752) ccw
  line L1187 (41.7928, 17.4945) -> (41.6245, 17.6628)
  arc A3398 (41.6805, 17.3823) -> (41.905, 17.6068) centre (41.7928, 17.4945) ccw
  arc A3399 (41.7368, 17.775) -> (41.5123, 17.5505) centre (41.6246, 17.6627) ccw
  line L1188 (40.64, 18.0213) -> (40.64, 16.51)
  line L1189 (26.94, 18.0065) -> (26.67, 17.7365)
  arc A3400 (26.5577, 17.8488) -> (26.7823, 17.6243) centre (26.67, 17.7366) ccw
  arc A3401 (39.4373, 17.4446) -> (39.6619, 17.6692) centre (39.5496, 17.5569) ccw
  arc A3402 (41.8991, 17.0181) -> (42.182, 17.1622) centre (42.0406, 17.0902) ccw
  line L1190 (29.21, 17.7365) -> (28.94, 18.0065)
  arc A3403 (41.5312, 17.5343) -> (41.7179, 17.7912) centre (41.6246, 17.6628) ccw
  arc A3404 (34.1777, 17.8488) -> (34.4023, 17.6243) centre (34.29, 17.7366) ccw
  arc A3405 (34.6723, 17.8943) -> (34.4478, 18.1188) centre (34.5601, 18.0066) ccw
  arc A3406 (27.6496, 18.1286) -> (27.5281, 18.422) centre (27.5889, 18.2753) ccw
  arc A3407 (40.5211, 18.18) -> (40.5211, 17.8625) centre (40.5211, 18.0212) ccw
  arc A3408 (40.0108, 18.0616) -> (40.1089, 17.7596) centre (40.0599, 17.9106) ccw
  arc A3409 (41.5254, 17.931) -> (41.3388, 17.6741) centre (41.4321, 17.8026) ccw
  arc A3410 (41.2922, 18.052) -> (41.1481, 17.7691) centre (41.2202, 17.9106) ccw
  arc A3411 (39.0392, 17.8599) -> (39.1607, 18.1532) centre (39.1, 18.0065) ccw
  arc A3412 (37.0393, 18.1532) -> (37.1608, 17.8599) centre (37.1, 18.0065) ccw
  arc A3413 (40.7589, 17.8625) -> (40.7589, 18.18) centre (40.7589, 18.0212) ccw
  arc A3414 (40.7987, 18.0213) -> (40.4812, 18.0213) centre (40.6399, 18.0213) ccw
  line L1191 (41.4321, 17.8026) -> (41.2201, 17.9106)
  arc A3415 (39.2122, 18.1188) -> (38.9877, 17.8943) centre (39.1, 18.0065) ccw
  line L1192 (41.9326, 17.3021) -> (41.7928, 17.4945)
  line L1193 (31.75, 17.7365) -> (31.48, 18.0065)
  line L1194 (39.5496, 17.5569) -> (39.1, 18.0065)
  arc A3416 (41.36, 17.6611) -> (41.5042, 17.944) centre (41.4321, 17.8026) ccw
  arc A3417 (41.1711, 17.7596) -> (41.2692, 18.0616) centre (41.2202, 17.9106) ccw
  arc A3418 (32.6689, 18.434) -> (32.6689, 18.1165) centre (32.6689, 18.2752) ccw
  line L1195 (37.1, 18.0065) -> (36.83, 17.7365)
  line L1196 (41.6245, 17.6628) -> (41.4321, 17.8026)
  arc A3419 (37.8096, 18.1286) -> (37.6881, 18.422) centre (37.7489, 18.2753) ccw
  line L1197 (41.2201, 17.9106) -> (40.9939, 17.9841)
  line L1198 (40.0599, 17.9106) -> (39.8479, 17.8026)
  line L1199 (40.64, 18.0213) -> (40.5211, 18.0213)
  arc A3420 (40.4813, 16.51) -> (40.7988, 16.51) centre (40.6401, 16.51) ccw
  line L1200 (40.64, 16.51) -> (40.64, 18.0213)
  arc A3421 (42.074, 17.3742) -> (41.7911, 17.23) centre (41.9325, 17.3021) ccw
  arc A3422 (39.5621, 17.7912) -> (39.7488, 17.5343) centre (39.6555, 17.6627) ccw
  arc A3423 (31.4192, 17.8599) -> (31.5407, 18.1532) centre (31.4799, 18.0065) ccw
  line L1201 (39.8479, 17.8026) -> (39.6555, 17.6628)
  arc A3424 (36.7177, 17.8488) -> (36.9423, 17.6243) centre (36.83, 17.7366) ccw
  arc A3425 (41.043, 18.1351) -> (40.9448, 17.8331) centre (40.9939, 17.9841) ccw
  line L1202 (37.7489, 18.2753) -> (37.1, 18.0065)
  line L1203 (38.4511, 18.2753) -> (37.7489, 18.2753)
  arc A3426 (39.7677, 17.5505) -> (39.5432, 17.775) centre (39.6555, 17.6627) ccw
  arc A3427 (40.64, 18.18) -> (40.64, 17.8625) centre (40.64, 18.0212) ccw
  arc A3428 (40.7988, 18.0213) -> (40.4813, 18.0213) centre (40.6401, 18.0213) ccw
  arc A3429 (38.5119, 18.422) -> (38.3904, 18.1286) centre (38.4511, 18.2753) ccw
  arc A3430 (40.64, 16.3513) -> (40.64, 16.6688) centre (40.64, 16.51) ccw
  arc A3431 (40.5459, 17.8645) -> (40.4962, 18.1781) centre (40.5211, 18.0213) ccw
  arc A3432 (40.2613, 18.1409) -> (40.3109, 17.8273) centre (40.2861, 17.9841) ccw
  line L1204 (40.9939, 17.9841) -> (40.7589, 18.0213)
  arc A3433 (41.9212, 17.5879) -> (41.6643, 17.4012) centre (41.7927, 17.4945) ccw
  arc A3434 (40.9691, 17.8273) -> (41.0187, 18.1409) centre (40.9939, 17.9841) ccw
  line L1205 (35.9111, 18.2753) -> (35.2089, 18.2753)
  arc A3435 (27.5889, 18.434) -> (27.5889, 18.1165) centre (27.5889, 18.2752) ccw
  arc A3436 (26.5577, 17.6243) -> (26.7823, 17.8488) centre (26.67, 17.7366) ccw
  arc A3437 (29.0522, 18.1188) -> (28.8277, 17.8943) centre (28.94, 18.0065) ccw
  arc A3438 (30.8311, 18.1165) -> (30.8311, 18.434) centre (30.8311, 18.2752) ccw
  arc A3439 (36.7177, 17.6243) -> (36.9423, 17.8488) centre (36.83, 17.7366) ccw
  arc A3440 (36.6722, 18.1188) -> (36.4477, 17.8943) centre (36.56, 18.0066) ccw
  arc A3441 (29.0977, 17.8488) -> (29.3223, 17.6243) centre (29.21, 17.7366) ccw
  arc A3442 (28.3519, 18.422) -> (28.2304, 18.1286) centre (28.2911, 18.2753) ccw
  arc A3443 (33.9592, 17.8599) -> (34.0807, 18.1532) centre (34.02, 18.0065) ccw
  arc A3444 (33.4319, 18.422) -> (33.3104, 18.1286) centre (33.3712, 18.2753) ccw
  line L1206 (31.48, 18.0065) -> (30.8311, 18.2753)
  line L1207 (26.67, 17.7365) -> (26.4, 18.0065)
  line L1208 (28.94, 18.0065) -> (28.2911, 18.2753)
  line L1209 (32.6689, 18.2753) -> (32.02, 18.0065)
  arc A3445 (32.1323, 17.8943) -> (31.9078, 18.1188) centre (32.0201, 18.0066) ccw
  line L1210 (28.2911, 18.2753) -> (27.5889, 18.2753)
  arc A3446 (31.9593, 18.1532) -> (32.0808, 17.8599) centre (32.0201, 18.0066) ccw
  arc A3447 (34.1322, 18.1188) -> (33.9077, 17.8943) centre (34.02, 18.0066) ccw
  arc A3448 (35.2089, 18.434) -> (35.2089, 18.1165) centre (35.2089, 18.2752) ccw
  arc A3449 (26.8793, 18.1532) -> (27.0008, 17.8599) centre (26.9401, 18.0065) ccw
  line L1211 (34.29, 17.7365) -> (34.02, 18.0065)
  arc A3450 (32.7296, 18.1286) -> (32.6081, 18.422) centre (32.6688, 18.2753) ccw
  arc A3451 (30.1896, 18.1286) -> (30.0681, 18.422) centre (30.1288, 18.2753) ccw
  arc A3452 (30.8919, 18.422) -> (30.7704, 18.1286) centre (30.8312, 18.2753) ccw
  line L1212 (34.56, 18.0065) -> (34.29, 17.7365)
  arc A3453 (29.5923, 17.8943) -> (29.3678, 18.1188) centre (29.4801, 18.0066) ccw
  line L1213 (30.1289, 18.2753) -> (29.48, 18.0065)
  line L1214 (29.48, 18.0065) -> (29.21, 17.7365)
  line L1215 (36.83, 17.7365) -> (36.56, 18.0065)
  arc A3454 (35.9111, 18.1165) -> (35.9111, 18.434) centre (35.9111, 18.2752) ccw
  arc A3455 (35.9719, 18.422) -> (35.8504, 18.1286) centre (35.9112, 18.2753) ccw
  arc A3456 (33.3711, 18.1165) -> (33.3711, 18.434) centre (33.3711, 18.2752) ccw
  line L1216 (35.2089, 18.2753) -> (34.56, 18.0065)
  arc A3457 (26.5122, 18.1188) -> (26.2877, 17.8943) centre (26.4, 18.0066) ccw
  arc A3458 (34.1777, 17.6243) -> (34.4023, 17.8488) centre (34.29, 17.7366) ccw
  line L1217 (34.02, 18.0065) -> (33.3711, 18.2753)
  arc A3459 (16.3815, 13.6963) -> (16.26, 13.9897) centre (16.3208, 13.843) ccw
  arc A3460 (31.6377, 17.8488) -> (31.8623, 17.6243) centre (31.75, 17.7366) ccw
  line L1218 (15.9006, 13.669) -> (15.5791, 13.3475)
  line L1219 (27.5889, 18.2753) -> (26.94, 18.0065)
  arc A3461 (15.4669, 13.4597) -> (15.6914, 13.2352) centre (15.5792, 13.3475) ccw
  arc A3462 (28.2911, 18.1165) -> (28.2911, 18.434) centre (28.2911, 18.2752) ccw
  line L1220 (21.3635, 15.51) -> (21.717, 15.1565)
  line L1221 (36.56, 18.0065) -> (35.9111, 18.2753)
  arc A3463 (28.8792, 17.8599) -> (29.0007, 18.1532) centre (28.94, 18.0065) ccw
  line L1222 (32.02, 18.0065) -> (31.75, 17.7365)
  line L1223 (26.4, 18.0065) -> (25.7511, 18.2753)
  arc A3464 (31.6377, 17.6243) -> (31.8623, 17.8488) centre (31.75, 17.7366) ccw
  arc A3465 (29.4193, 18.1532) -> (29.5408, 17.8599) centre (29.4801, 18.0065) ccw
  line L1224 (30.8311, 18.2753) -> (30.1289, 18.2753)
  arc A3466 (36.4992, 17.8599) -> (36.6207, 18.1532) centre (36.56, 18.0065) ccw
  arc A3467 (35.2696, 18.1286) -> (35.1481, 18.422) centre (35.2088, 18.2753) ccw
  arc A3468 (27.0523, 17.8943) -> (26.8278, 18.1188) centre (26.9401, 18.0066) ccw
  arc A3469 (29.0977, 17.6243) -> (29.3223, 17.8488) centre (29.21, 17.7366) ccw
  arc A3470 (30.1289, 18.434) -> (30.1289, 18.1165) centre (30.1289, 18.2752) ccw
  arc A3471 (31.5922, 18.1188) -> (31.3677, 17.8943) centre (31.4799, 18.0066) ccw
  line L1225 (33.3711, 18.2753) -> (32.6689, 18.2753)
  arc A3472 (34.4993, 18.1532) -> (34.6208, 17.8599) centre (34.5601, 18.0065) ccw
  arc A3473 (25.7511, 18.1165) -> (25.7511, 18.434) centre (25.7511, 18.2752) ccw
  arc A3474 (23.9722, 18.1188) -> (23.7477, 17.8943) centre (23.86, 18.0065) ccw
  line L1226 (25.0489, 18.2753) -> (24.4, 18.0065)
  arc A3475 (16.0129, 13.5567) -> (15.7884, 13.7812) centre (15.9007, 13.6689) ccw
  line L1227 (21.0947, 16.8611) -> (21.0947, 16.1589)
  arc A3476 (21.9723, 17.8943) -> (21.7478, 18.1188) centre (21.8601, 18.0066) ccw
  arc A3477 (21.7993, 18.1532) -> (21.9208, 17.8599) centre (21.8601, 18.0065) ccw
  arc A3478 (23.2111, 18.1165) -> (23.2111, 18.434) centre (23.2111, 18.2752) ccw
  line L1228 (14.6499, 12.9032) -> (13.7795, 12.0328)
  arc A3479 (25.8119, 18.422) -> (25.6904, 18.1286) centre (25.7512, 18.2753) ccw
  line L1229 (21.0947, 16.1589) -> (21.3635, 15.51)
  arc A3480 (21.2535, 16.8611) -> (20.9359, 16.8611) centre (21.0947, 16.8611) ccw
  arc A3481 (15.6914, 13.2352) -> (15.4669, 13.4597) centre (15.5792, 13.3475) ccw
  arc A3482 (21.5101, 17.4492) -> (21.2168, 17.5707) centre (21.3635, 17.5099) ccw
  arc A3483 (24.3393, 18.1532) -> (24.4608, 17.8599) centre (24.4001, 18.0065) ccw
  arc A3484 (21.2414, 16.2196) -> (20.948, 16.0981) centre (21.0947, 16.1589) ccw
  line L1230 (23.86, 18.0065) -> (23.2111, 18.2753)
  line L1231 (21.1166, 13.843) -> (16.3207, 13.843)
  arc A3485 (22.5696, 18.1286) -> (22.4481, 18.422) centre (22.5089, 18.2753) ccw
  line L1232 (21.86, 18.0065) -> (21.3635, 17.51)
  arc A3486 (21.8758, 15.1565) -> (21.5583, 15.1565) centre (21.717, 15.1565) ccw
  line L1233 (21.717, 14.4434) -> (21.1166, 13.843)
  arc A3487 (23.2719, 18.422) -> (23.1504, 18.1286) centre (23.2111, 18.2753) ccw
  arc A3488 (22.5089, 18.434) -> (22.5089, 18.1165) centre (22.5089, 18.2752) ccw
  line L1234 (15.5791, 13.3475) -> (15.1349, 12.9032)
  arc A3489 (13.6672, 12.145) -> (13.8918, 11.9205) centre (13.7795, 12.0328) ccw
  arc A3490 (20.948, 16.9219) -> (21.2414, 16.8004) centre (21.0947, 16.8612) ccw
  arc A3491 (13.6208, 10.8018) -> (13.9383, 10.8018) centre (13.7796, 10.8018) ccw
  line L1235 (24.13, 17.7365) -> (23.86, 18.0065)
  line L1236 (21.3635, 17.51) -> (21.0947, 16.8611)
  arc A3492 (21.0043, 13.9553) -> (21.2288, 13.7307) centre (21.1165, 13.843) ccw
  arc A3493 (21.5583, 14.4434) -> (21.8758, 14.4434) centre (21.717, 14.4434) ccw
  arc A3494 (21.8293, 14.3312) -> (21.6047, 14.5557) centre (21.717, 14.4435) ccw
  arc A3495 (21.2168, 15.4493) -> (21.5101, 15.5708) centre (21.3635, 15.51) ccw
  arc A3496 (23.7992, 17.8599) -> (23.9207, 18.1532) centre (23.8599, 18.0065) ccw
  line L1237 (22.5089, 18.2753) -> (21.86, 18.0065)
  arc A3497 (25.0489, 18.434) -> (25.0489, 18.1165) centre (25.0489, 18.2752) ccw
  arc A3498 (24.0177, 17.8488) -> (24.2423, 17.6243) centre (24.13, 17.7366) ccw
  arc A3499 (15.1349, 12.7444) -> (15.1349, 13.0619) centre (15.1349, 12.9032) ccw
  arc A3500 (21.4757, 15.6223) -> (21.2512, 15.3978) centre (21.3635, 15.51) ccw
  arc A3501 (15.8399, 13.8157) -> (15.9614, 13.5223) centre (15.9007, 13.669) ccw
  arc A3502 (14.6499, 13.0619) -> (14.6499, 12.7444) centre (14.6499, 12.9032) ccw
  arc A3503 (24.0177, 17.6243) -> (24.2423, 17.8488) centre (24.13, 17.7366) ccw
  line L1238 (24.4, 18.0065) -> (24.13, 17.7365)
  arc A3504 (20.9359, 16.1589) -> (21.2535, 16.1589) centre (21.0947, 16.1589) ccw
  arc A3505 (26.3392, 17.8599) -> (26.4607, 18.1532) centre (26.3999, 18.0065) ccw
  arc A3506 (15.0226, 13.0155) -> (15.2471, 12.7909) centre (15.1349, 12.9032) ccw
  line L1239 (21.717, 15.1565) -> (21.717, 14.4434)
  line L1240 (25.7511, 18.2753) -> (25.0489, 18.2753)
  arc A3507 (14.7622, 12.7909) -> (14.5377, 13.0155) centre (14.65, 12.9032) ccw
  arc A3508 (25.1096, 18.1286) -> (24.9881, 18.422) centre (25.0489, 18.2753) ccw
  arc A3509 (21.2512, 17.6222) -> (21.4757, 17.3977) centre (21.3635, 17.5099) ccw
  line L1241 (13.7795, 12.0328) -> (13.7795, 10.8018)
  line L1242 (23.2111, 18.2753) -> (22.5089, 18.2753)
  line L1243 (15.1349, 12.9032) -> (14.6499, 12.9032)
  arc A3510 (24.5123, 17.8943) -> (24.2878, 18.1188) centre (24.4001, 18.0066) ccw
  arc A3511 (65.9384, 2.7686) -> (65.9384, 2.7178) centre (65.9384, 2.7432) ccw
  arc A3512 (66.0553, 2.2782) -> (66.0811, 2.2345) centre (66.0682, 2.2564) ccw
  arc A3513 (63.0301, 1.5494) -> (63.0301, 1.6002) centre (63.0301, 1.5748) ccw
  arc A3514 (57.5748, 1.5748) -> (57.6256, 1.5748) centre (57.6002, 1.5748) ccw
  arc A3515 (66.1981, 2.4836) -> (65.9384, 2.7432) centre (65.9384, 2.4835) ccw
  arc A3516 (65.556, 1.8344) -> (65.6068, 1.8344) centre (65.5814, 1.8344) ccw
  arc A3517 (58.2027, 1.5748) -> (58.2535, 1.5748) centre (58.2281, 1.5748) ccw
  line L1244 (55.3077, 1.5748) -> (55.827, 1.5748)
  arc A3518 (55.4375, 2.2493) -> (55.4375, 2.1985) centre (55.4375, 2.2239) ccw
  arc A3519 (65.1543, 2.4836) -> (65.1035, 2.4836) centre (65.1289, 2.4836) ccw
  arc A3520 (58.9026, 2.7432) -> (58.8518, 2.7432) centre (58.8772, 2.7432) ccw
  arc A3521 (55.8524, 2.7432) -> (55.8016, 2.7432) centre (55.827, 2.7432) ccw
  arc A3522 (63.0142, 2.4637) -> (63.046, 2.5034) centre (63.0301, 2.4835) ccw
  line L1245 (54.5067, 2.0941) -> (54.8313, 2.0941)
  arc A3523 (56.6617, 1.5668) -> (56.7099, 1.5828) centre (56.6858, 1.5748) ccw
  arc A3524 (61.238, 1.6002) -> (61.238, 1.5494) centre (61.238, 1.5748) ccw
  line L1246 (57.73, 1.5748) -> (57.4703, 1.5748)
  arc A3525 (55.827, 2.1985) -> (55.827, 2.2493) centre (55.827, 2.2239) ccw
  arc A3526 (54.1594, 1.5862) -> (54.2049, 1.5634) centre (54.1822, 1.5748) ccw
  arc A3527 (55.3077, 1.6002) -> (55.3077, 1.5494) centre (55.3077, 1.5748) ccw
  arc A3528 (54.8313, 2.0687) -> (54.8313, 2.1195) centre (54.8313, 2.0941) ccw
  line L1247 (55.827, 1.5748) -> (55.827, 2.7432)
  arc A3529 (63.524, 1.6002) -> (63.524, 1.5494) centre (63.524, 1.5748) ccw
  arc A3530 (66.2234, 2.4836) -> (66.1727, 2.4836) centre (66.1981, 2.4836) ccw
  arc A3531 (65.6311, 2.6662) -> (65.6615, 2.6255) centre (65.6463, 2.6459) ccw
  line L1248 (59.4473, 1.8994) -> (59.4473, 2.7432)
  arc A3532 (56.6617, 1.5828) -> (56.7099, 1.5668) centre (56.6858, 1.5748) ccw
  arc A3533 (53.11, 1.8344) -> (53.0592, 1.8344) centre (53.0846, 1.8344) ccw
  arc A3534 (53.0846, 1.8344) -> (53.3443, 1.5748) centre (53.3443, 1.8345) ccw
  arc A3535 (66.0804, 2.2341) -> (66.0561, 2.2787) centre (66.0682, 2.2564) ccw
  line L1249 (58.8772, 2.7432) -> (58.2281, 1.5748)
  arc A3536 (53.3443, 1.5494) -> (53.3443, 1.6002) centre (53.3443, 1.5748) ccw
  line L1250 (54.1822, 1.5748) -> (54.4418, 2.0941)
  arc A3537 (57.0993, 2.7352) -> (57.0511, 2.7512) centre (57.0752, 2.7432) ccw
  arc A3538 (53.3443, 1.5748) -> (53.7337, 1.7371) centre (53.3442, 2.1232) ccw
  line L1251 (57.0752, 2.7432) -> (56.6858, 1.5748)
  line L1252 (56.6858, 1.5748) -> (56.2963, 2.7432)
  arc A3539 (64.1731, 1.5494) -> (64.1731, 1.6002) centre (64.1731, 1.5748) ccw
  line L1253 (61.8871, 2.4836) -> (61.5626, 2.7432)
  arc A3540 (61.8871, 1.5494) -> (61.8871, 1.6002) centre (61.8871, 1.5748) ccw
  line L1254 (65.1289, 1.8344) -> (65.1289, 2.4836)
  arc A3541 (54.4645, 2.0827) -> (54.4191, 2.1054) centre (54.4418, 2.0941) ccw
  line L1255 (55.827, 2.2239) -> (55.4375, 2.2239)
  arc A3542 (53.3443, 1.6002) -> (53.3443, 1.5494) centre (53.3443, 1.5748) ccw
  arc A3543 (64.1572, 2.4637) -> (64.189, 2.5034) centre (64.1731, 2.4835) ccw
  line L1256 (64.1731, 1.5748) -> (63.524, 1.5748)
  arc A3544 (66.2485, 1.7192) -> (66.2125, 1.755) centre (66.2305, 1.7371) ccw
  arc A3545 (65.1543, 1.8344) -> (65.1035, 1.8344) centre (65.1289, 1.8344) ccw
  line L1257 (64.8693, 2.7432) -> (64.6096, 2.7432)
  arc A3546 (64.8693, 1.5748) -> (65.1289, 1.8344) centre (64.8693, 1.8344) ccw
  arc A3547 (63.8644, 2.763) -> (63.8327, 2.7234) centre (63.8485, 2.7432) ccw
  arc A3548 (65.1289, 2.4836) -> (64.8693, 2.7432) centre (64.8693, 2.4836) ccw
  arc A3549 (63.8232, 1.5748) -> (63.874, 1.5748) centre (63.8486, 1.5748) ccw
  arc A3550 (66.0682, 2.2564) -> (66.1981, 2.4836) centre (65.9344, 2.4836) ccw
  arc A3551 (62.381, 1.6002) -> (62.381, 1.5494) centre (62.381, 1.5748) ccw
  arc A3552 (61.5372, 1.5748) -> (61.588, 1.5748) centre (61.5626, 1.5748) ccw
  arc A3553 (61.5784, 2.763) -> (61.5467, 2.7234) centre (61.5625, 2.7432) ccw
  line L1258 (60.0964, 2.7432) -> (60.0964, 1.8994)
  arc A3554 (65.9384, 2.7432) -> (65.6463, 2.6458) centre (65.9384, 2.2564) ccw
  line L1259 (61.5626, 2.7432) -> (61.5626, 1.5748)
  arc A3555 (54.5067, 2.1195) -> (54.5067, 2.0687) centre (54.5067, 2.0941) ccw
  line L1260 (58.2281, 1.5748) -> (58.2281, 2.7432)
  arc A3556 (57.4703, 1.6002) -> (57.4703, 1.5494) centre (57.4703, 1.5748) ccw
  line L1261 (65.7112, 2.0616) -> (66.0682, 2.2564)
  arc A3557 (64.8693, 2.7178) -> (64.8693, 2.7686) centre (64.8693, 2.7432) ccw